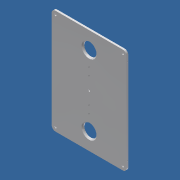
# Autodesk Inventor part: J001395
Saved by Autodesk Inventor 2012 SP2 (Build 160219200, 219)
## iProperties
Created: 2012-04-17
Part Number: J001395
Material: ALUMINUM, 6061-T651
Vendor: HHMI: JFRC - ID&F
Document SubType Name: Modeling
Designer: NEGRASHOVI
Density: 2.7 g/cm^3
Project: P-51601
Mass: 1484.19 g
Surface Area: 1842.91 cm^2
Volume: 549.698 cm^3
Description: HEATER PLATE
RuleStatus: InUse
AfterDocSave0: file://Part Number Cleaner
LAB/DEPT: GONEN (LAB)
REQUESTING SCIENTIST: GONEN, TAMIR
SURFACE ROUGHNESS: 32 Ra
DESIGN DEPARTMENT: HHMI: JFRC - ID&F
SPECIAL FINISH: ANODIZE PER MIL-A-8625F, TYPE II, CLASS 2 (BLACK)
ALTERED ITEM PART NUMBER: N/A
ALTERED ITEM VENDOR: N/A
ALTERED ITEM DESCRIPTION: N/A
Author: NEGRASHOVI
Revision Number: -
Autodesk Inventor part; units mm, degrees
ref_plane "YZ Plane" through (0, 0, 0) normal (1, 0, 0) x (0, 1, 0)
ref_plane "XZ Plane" through (0, 0, 0) normal (0, 1, 0) x (-1, 0, 0)
ref_plane "XY Plane" through (0, 0, 0) normal (0, 0, 1) x (1, 0, 0)
sketch "Sketch1" plane through (0, 0, 0) normal (0, 0, 1) x (1, 0, 0)
  line L0 (-127, 177.8) -> (127, 177.8)
  line L1 (127, 177.8) -> (127, -177.8)
  line L2 (127, -177.8) -> (-127, -177.8)
  line L3 (-127, -177.8) -> (-127, 177.8)
  point P0 (0, 0)
  dimension "d0" = 254
  dimension "d1" = 127
  dimension "d2" = 355.6
  dimension "d3" = 177.8
  constraints: 8 end point, 2 parallel, 1 horizontal, 1 perpendicular
  measures "d0" distance of L0.start L0.end
  measures "d1" distance from line of L3 point (0, 0)
  measures "d2" distance of L0.end L1.end
  measures "d3" distance from line of point (0, 0) L0
extrude "Extrusion1" add sketch "Sketch1" along normal blind 6.35
sketch "Sketch2" plane through (0, 0, 6.35) normal (0, 0, 1) x (1, 0, 0)
  line L0 (-114.3, 165.1) -> (114.3, 165.1) construction
  line L1 (114.3, 165.1) -> (114.3, -165.1) construction
  line L2 (114.3, -165.1) -> (-114.3, -165.1) construction
  line L3 (-114.3, -165.1) -> (-114.3, 165.1) construction
  line L4 (-127, 177.8) -> (127, 177.8) construction
  line L5 (127, -177.8) -> (-127, -177.8) construction
  line L6 (-127, -177.8) -> (-127, 177.8) construction
  line L7 (127, 177.8) -> (127, -177.8) construction
  point P0 (0, 0)
  point P1 (0, 0)
  dimension "d6" = 12.7
  dimension "d7" = 12.7
  dimension "d8" = 12.7
  dimension "d9" = 12.7
  constraints: 8 end point, 5 coincident, 2 parallel, 1 horizontal, 1 perpendicular
  measures "d6" distance between parallel lines of L0 L4
  measures "d7" distance between parallel lines of L5 L2
  measures "d8" distance between parallel lines of L6 L3
  measures "d9" distance between parallel lines of L1 L7
hole "Hole1" at (-114.3, 165.1, 6.35) at (114.3, 165.1, 6.35) at (114.3, -165.1, 6.35) at (-114.3, -165.1, 6.35) at (0, 0, 6.35) direction (0, 0, -1) diameter 6.7564 end through all clearance for "Flat Head Machine Screw (82)" size "1/4" standard "Ansi Unified Screw Threads"
sketch "Sketch3" plane through (0, 0, 6.35) normal (0, 0, 1) x (1, 0, 0)
  line L0 (0, 248.92) -> (0, -248.92) construction
  point P0 (0, 0)
  point P1 (0, 119.38)
  point P2 (0, -119.38)
  dimension "d17" = 238.76
  dimension "d18" = 119.38
  constraints: 2 point on line
  measures "d17" distance of point (0, -119.38) point (0, 119.38)
  measures "d18" distance of point (0, 0) point (0, 119.38)
hole "Hole2" at (0, 119.38, 6.35) at (0, -119.38, 6.35) direction (0, 0, -1) diameter 44.45 end through all
sketch "Sketch4" plane through (0, 0, 6.35) normal (0, 0, 1) x (1, 0, 0)
  line L0 (0, -248.92) -> (0, 248.92) construction
  circle A0 centre (0, 119.38) radius 22.225 construction
  circle A1 centre (0, -119.38) radius 22.225 construction
  line L1 (-177.8, 0) -> (177.8, 0) construction
  point P0 (0, 0)
  point P1 (0, 68.58)
  point P2 (0, 43.18)
  point P3 (0, -68.58)
  point P4 (0, -43.18)
  dimension "d26" = 50.8
  dimension "d27" = 25.4
  dimension "d28" = 50.8
  dimension "d29" = 25.4
  constraints: 4 point on line
  measures "d26" distance of point (0, 68.58) A0.centre
  measures "d27" distance of point (0, 43.18) point (0, 68.58)
  measures "d28" distance of point (0, -68.58) A1.centre
  measures "d29" distance of point (0, -43.18) point (0, -68.58)
hole "Hole3" at (0, 68.58, 6.35) at (0, 43.18, 6.35) at (0, -68.58, 6.35) at (0, -43.18, 6.35) direction (0, 0, -1) diameter 3.302 end through all thread size "8-32 UNC" class "2B" standard "ANSI Unified Screw Threads"
fillet "Fillet1" radius 12.7 4 edges at (127, -177.8, 3.175) (-127, -177.8, 3.175) (127, 177.8, 3.175) (-127, 177.8, 3.175)
chamfer "Chamfer1" distance 3.175 angle 45 2 edges at (0, -97.155, 6.35) (0, 141.605, 6.35)
sketch "Sketch6" plane through (127, -165.1, 0) normal (1, 0, 0) x (0, 0, -1)
  line L0 (-6.35, 330.2) -> (0, 330.2) projected
  line L1 (-6.35, 330.2) -> (-6.35, 0) projected
  line L2 (0, 0) -> (-6.35, 0) projected
  line L3 (0, 330.2) -> (0, 0) projected
  line L4 (-3.175, 330.2) -> (-3.175, 0) construction
  line L5 (0, 165.1) -> (-6.35, 165.1) construction
  point P0 (-3.175, 165.1)
  point P1 (-3.175, 311.15)
  point P2 (-3.175, 19.05)
  dimension "d52" = 146.05
  constraints: 4 end point, 4 midpoint, 2 point on line, 1 symmetric about line
  measures "d52" distance of point (-3.175, 311.15) point (-3.175, 165.1)
hole "Hole5" at (127, 0, 3.175) at (127, 146.05, 3.175) at (127, -146.05, 3.175) direction (-1, 0, 0) diameter 2.6416 depth 15.24 tip angle 118 thread size "6-32 UNC" class "2B" standard "ANSI Unified Screw Threads"
mirror "Mirror1" about plane through (0, 0, 0) normal (1, 0, 0) of "Hole5"
equation "\"d1\" = 0.5 * d0"
equation "\"d3\" = 0.5 * d2"
equation "\"d18\" = 0.5 * d17"
body "Solid1"
